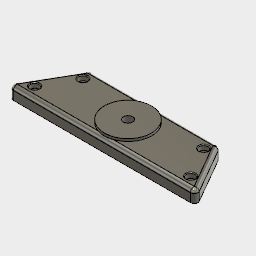
FootMount v1 (Autodesk Fusion 360 design; units mm, degrees)
Autodesk Fusion 360 part; units mm, degrees
note: some values were not read from the file. Chosen so that the rebuilt part matches the saved one: which face or edge a step refers to. Set by a fixed rule: which sketch regions a step uses.
sketch "Sketch1" plane through (0, 0, 0) normal (0, 1, 0) x (1, 0, 0)
  line L0 (0, 0) -> (153, 0)
  line L1 (153, 0) -> (153, 42)
  line L2 (153, 42) -> (0, 42)
  line L3 (0, 42) -> (0, 0)
  line L4 (76.5, 42) -> (124, 42)
  line L5 (153, 0) -> (128.7513, 42)
  line L6 (153, 0) -> (201.4974, 0) construction
  line L7 (76.5, 0) -> (76.5, 42)
  line L8 (0, 0) -> (24.2487, 42)
  dimension "d1" = 42
  dimension "d2" = 120
  measures "d1" distance of L0.start L2.end
  measures "d2" angle of L5 L6
extrude "Extrude1" add sketch "Sketch1" along normal blind 10 contours L0 L2 L7 L8 | L0 L2 L4 L5 L7 makes body 1
fillet "Fillet1" radius 3 11 edges at (100.25, 10, -42) (24.2487, 5, -42) (50.3744, 10, -42) (0, 5, 0) (12.1244, 10, -21) (38.25, 10, 0) (153, 5, 0) (114.75, 10, 0) (128.7513, 5, -42) (140.8756, 10, -21) (126.3756, 10, -42) on bodies 1
sketch "Sketch2" plane through (0, 10, 0) normal (0, 1, 0) x (-1, 0, 0)
  line L0 (-147.8038, -3) -> (-127.0192, -39)
  line L1 (-127.0192, -39) -> (-25.9808, -39)
  line L2 (-25.9808, -39) -> (-5.1962, -3)
  line L3 (-5.1962, -3) -> (-147.8038, -3)
  line L4 (-76.5, -39) -> (-76.5, -3)
  circle A0 centre (-76.5, -21) radius 3.75
  circle A1 centre (-76.5, -21) radius 19
  dimension "d6" = 7.5
  dimension "d7" = 38
  measures "d6" diameter of A0
  measures "d7" diameter of A1
extrude "Extrude2" add sketch "Sketch2" against normal blind 6 contours L3 A1 | L1 L3 L4 A0 A1 | L1 A1 | L1 L3 L4 A0 A1 bodies 1
extrude "Extrude3" add sketch "Sketch2" along normal blind 2 contours L3 A1 | L1 L3 L4 A0 A1 | L1 A1 | L1 L3 L4 A0 A1 bodies 1
extrude "Extrude4" cut sketch "Sketch2" against normal blind 8 contours L4 A0 | L4 A0 bodies 1
sketch "Sketch3" plane through (0, 0, 0) normal (0, -1, 0) x (1, 0, 0)
  arc A0 (127.0192, -42) -> (129.6173, -40.5) centre (127.0192, -39) ccw
  line L0 (129.6173, -40.5) -> (150.4019, -4.5)
  arc A1 (150.4019, -4.5) -> (147.8038, 0) centre (147.8038, -3) ccw
  line L1 (147.8038, 0) -> (5.1962, 0)
  arc A2 (5.1962, 0) -> (2.5981, -4.5) centre (5.1962, -3) ccw
  line L2 (2.5981, -4.5) -> (23.3827, -40.5)
  arc A3 (23.3827, -40.5) -> (25.9808, -42) centre (25.9808, -39) ccw
  line L3 (25.9808, -42) -> (127.0192, -42)
  line L4 (76.5, 0) -> (76.5, -42)
  line L5 (20.7846, -21) -> (45.0333, -21) construction
  line L6 (20.7846, -21) -> (45.0333, -21) construction
  circle A4 centre (13.6603, -8.6603) radius 1.75
  circle A5 centre (13.6603, -8.6603) radius 3.5
  circle A6 centre (27.909, -33.3397) radius 1.75
  circle A7 centre (27.909, -33.3397) radius 3.5
  circle A8 centre (139.3397, -8.6603) radius 3.5
  circle A9 centre (139.3397, -8.6603) radius 1.75
  circle A10 centre (125.091, -33.3397) radius 3.5
  circle A11 centre (125.091, -33.3397) radius 1.75
  point P0 (76.5, -21)
  point P1 (20.7846, -21)
  dimension "d18" = 3.5
  dimension "d19" = 7
  dimension "d20" = 3.5
  dimension "d21" = 7
  measures "d18" diameter of A4
  measures "d19" diameter of A5
  measures "d20" diameter of A6
  measures "d21" diameter of A7
extrude "Extrude5" cut sketch "Sketch3" against normal blind 15 contours A4 | A5 | A7 | A8 | A9 | A10 | A11 bodies 1 makes body 2 at (29.4022, 3.3333, -34.2523)
extrude "Extrude6" cut 1 faces at (28.68, 0, -32.758) along direction (0, 1, 0) blind 15 on bodies 2 bodies 2
extrude "Extrude7" add sketch "Sketch3" against normal blind 6 contours A5 | A7 | A8 | A10 bodies 1 2
fillet "Fillet2" radius 0.6 4 edges at (10.3971, 10, -9.9259) (24.6458, 10, -34.6054) (136.0766, 10, -9.9259) (121.8279, 10, -34.6054) on bodies 1
copy_body "Body->Comp1" bodies 1 removing the originals makes body 3 in component "FootMount"
component "FootMount" placed x (1, 0, 0) y (0, 1, 0) z (0, 0, 1) at (0, 0, 0)
